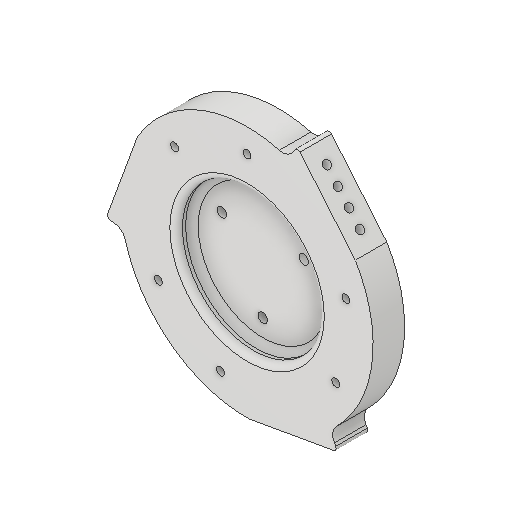
# Autodesk Inventor part: 3DP_ABS_Bowl_Springs_Mount_Plate
Saved by Autodesk Inventor 2025 (Build 290162010, 162A)
## iProperties
Created: 2018-05-26
Part Number: 3DP_ABS_Bowl_Springs_Mount_Plate
Material: ABS Plastic
Document SubType Name: Modeling
Designer: Andrzej
Density: 1.06 g/cm^3
Appearance: Smooth - White
Author: Andrzej
Autodesk Inventor part; units mm, degrees
ref_plane "YZ Plane" through (0, 0, 0) normal (1, 0, 0) x (0, 1, 0)
ref_plane "XZ Plane" through (0, 0, 0) normal (0, 1, 0) x (-1, 0, 0)
ref_plane "XY Plane" through (0, 0, 0) normal (0, 0, 1) x (1, 0, 0)
sketch "Sketch1" plane through (0, 0, 0) normal (0, 0, 1) x (1, 0, 0)
  circle A0 centre (0, 0) radius 40
  circle A1 centre (0, 0) radius 20
  dimension "d0" = 80
  dimension "d83" = 40
  constraints: 2 centre point, 2 coincident
  measures "d0" diameter of A0
  measures "d83" diameter of A1
extrude "Extrusion1" add sketch "Sketch1" along normal blind 10 contours A0 | A1
sketch "Sketch3" plane through (0, 0, 0) normal (0, 0, -1) x (-1, 0, 0)
  circle A0 centre (0, 0) radius 40 projected
  line L0 (44.7501, -7.5) -> (39.2906, 7.5)
  line L1 (44.7501, -7.5) -> (95.2438, -7.5) construction
  line L2 (44.7501, -7.5) -> (39.2906, -7.5)
  circle A1 centre (0, 0) radius 40 projected
  line L3 (39.2906, 7.5) -> (34.9192, 19.5102)
  dimension "d16" = 110
  dimension "d17" = 7.5
  dimension "d18" = 7.5
  constraints: 8 end point, 3 point on circle, 2 horizontal, 1 collinear
  measures "d16" angle of L1 L0
  measures "d17" distance from line of point (0, 0) L2
  measures "d18" vertical distance of point (0, 0) L0.end
extrude "Extrusion2" add sketch "Sketch3" against normal up to surface (10 mm away) contours A0 L0 L2
extrude "Extrusion3" cut sketch "Sketch3" against normal up to surface (10 mm away) contours L3 A0 picked at (37.4917, 12.8874)
fillet "Fillet1" radius 4 1 edges at (-39.2906, -7.5, 5)
fillet "Fillet1" radius 1 1 edges at (-44.7501, -7.5, 5)
sketch "Sketch4" plane through (-34.9192, 19.5102, 0) normal (-0.9396926, 0.3420201, 0) x (0, 0, 1)
  line L0 (10, -27.3155) -> (0, -27.3155) projected
  line L1 (10, -27.3155) -> (10, 0) projected
  line L2 (0, 0) -> (10, 0) projected
  line L3 (0, -27.3155) -> (0, 0) projected
  point P0 (0, -6.3905)
  point P1 (5, -5.4631)
  point P2 (5, -10.9262)
  point P3 (5, -16.3893)
  point P4 (5, -21.8524)
  dimension "d28" = 27.3155
  dimension "d29" = 5.4631
  dimension "d32" = 5.4631
  dimension "d44" = 10
  dimension "d45" = 5
  constraints: 1 vertical, 3 other
  measures "d28" distance between parallel lines of L0 L2
  measures "d29" distance from line of L2 point (5, -5.463)
  measures "d32" distance of point (5, -5.463) point (5, -10.926)
  measures "d44" distance of L2.start L1.end
  measures "d45" distance from line of L1 point (5, -5.463)
hole "Hole2" at (-36.7877, 14.3765, 5) at (-38.6562, 9.2429, 5) at (-40.5247, 4.1093, 5) at (-42.3932, -1.0244, 5) direction (0.9396926, -0.3420201, 0) diameter 2.5 depth 15 tip angle 118
pattern_circular "Circular Pattern2" count 3 over 360 about axis through (0, 0, 0) along (0, 0, 1) of "Extrusion2", "Extrusion3", "Fillet1", "Hole2"
sketch "Sketch7" plane through (0, 0, 10) normal (0, 0, 1) x (1, 0, 0)
  arc A0 (16.7979, 41.4107) -> (15.1658, 41.2679) centre (16.0318, 40.7679) ccw projected
  line L0 (14.7401, 40.5306) -> (15.1658, 41.2679) projected
  arc A1 (10.2509, 38.6642) -> (14.7401, 40.5306) centre (11.276, 42.5306) ccw projected
  arc A2 (10.2509, 38.6642) -> (-34.9192, 19.5102) centre (0, 0) ccw projected
  line L1 (-44.2617, -6.158) -> (-34.9192, 19.5102) projected
  arc A3 (-44.2617, -6.158) -> (-43.322, -7.5) centre (-43.322, -6.5) ccw projected
  line L2 (-42.4706, -7.5) -> (-43.322, -7.5) projected
  arc A4 (-38.6096, -10.4545) -> (-42.4706, -7.5) centre (-42.4706, -11.5) ccw projected
  arc A5 (-38.6096, -10.4545) -> (0.5633, -39.996) centre (0, 0) ccw projected
  line L3 (27.4638, -35.2528) -> (0.5633, -39.996) projected
  arc A6 (27.4638, -35.2528) -> (28.1562, -33.7679) centre (27.2902, -34.2679) ccw projected
  line L4 (27.7305, -33.0306) -> (28.1562, -33.7679) projected
  arc A7 (28.3587, -28.2096) -> (27.7305, -33.0306) centre (31.1946, -31.0306) ccw projected
  arc A8 (28.3587, -28.2096) -> (34.3559, 20.4859) centre (0, 0) ccw projected
  line L5 (16.7979, 41.4107) -> (34.3559, 20.4859) projected
  circle A9 centre (0, 0) radius 32.5
  line L6 (0, 0) -> (-22.981, 22.981)
  line L7 (0, 0) -> (35.2561, 0) construction
  point P0 (0, 32.5)
  dimension "d77" = 65
  dimension "d79" = 135
  constraints: 4 end point, 2 coincident, 2 point on circle, 1 centre point, 1 horizontal
  measures "d77" diameter of A9
  measures "d79" angle of L7 L6
hole "Hole4" at (0, 32.5, 10) at (-22.981, 22.981, 10) direction (0, 0, -1) diameter 2.5 end through all
pattern_circular "Circular Pattern5" count 3 over 360 about axis through (0, 0, -10) along (0, 0, 1) of "Hole4"
sketch "Sketch8" plane through (0, 0, 10) normal (0, 0, 1) x (1, 0, 0)
  circle A0 centre (0, 0) radius 22.5
  dimension "d84" = 45
  constraints: 1 centre point, 1 coincident
  measures "d84" diameter of A0
extrude "Extrusion4" cut sketch "Sketch8" against normal blind 5
fillet "Fillet2" radius 2 2 edges at (-22.5, 0, 5) (-22.5, 0, 10)
sketch "Sketch9" plane through (0, 0, 5) normal (0, 0, 1) x (1, 0, 0)
  point P0 (0, 0)
  point P1 (0, -15)
  point P2 (12.9904, 7.5)
  point P3 (-12.9904, 7.5)
  dimension "d88" = 15
  dimension "d91" = 360
  constraints: 4 other
  measures "d88" distance of point (0, 0) point (0, -15)
hole "Hole5" at (0, -15, 5) at (12.9904, 7.5, 5) at (-12.9904, 7.5, 5) direction (0, 0, -1) diameter 3 end through all
equation "\"d18\" = d17"
equation "\"d29\" = 0.2 * d28"
equation "\"d32\" = d29"
body "Solid1"
